New Bottom Plate_v1 (Autodesk Fusion 360 design; units mm, degrees)
Autodesk Fusion 360 part; units mm, degrees
sketch "Sketch1" plane through (0, 0, 0) normal (0, 0, 1) x (1, 0, 0)
  line L0 (0, 0) -> (342.375, 0)
  line L1 (342.375, 0) -> (342.375, 123.3)
  line L2 (342.375, 123.3) -> (0, 123.3)
  line L3 (0, 123.3) -> (0, 0)
  dimension "d1" = 342.375
  dimension "d2" = 123.3
  constraint horizontal L0
  constraint vertical L1
  constraint horizontal L2
  constraint vertical L3
  constraint coincident L0.start L3.end
  measures "d1" distance of L1.end L2.end
  measures "d2" distance of L0.start L2.end
extrude "Extrude1" add sketch "Sketch1" along normal blind 1
fillet "Fillet1" radius 2.5 4 edges at (0, 0, 0.5) (342.375, 0, 0.5) (342.375, 123.3, 0.5) (0, 123.3, 0.5)
sketch "Sketch2" plane through (0, 0, 1) normal (0, 0, 1) x (-1, 0, 0)
  arc A0 (-2.5, -123.3) -> (0, -120.8) centre (-2.5, -120.8) ccw
  line L0 (0, -120.8) -> (0, -2.5)
  arc A1 (0, -2.5) -> (-2.5, 0) centre (-2.5, -2.5) ccw
  line L1 (-2.5, 0) -> (-339.875, 0)
  arc A2 (-339.875, 0) -> (-342.375, -2.5) centre (-339.875, -2.5) ccw
  line L2 (-342.375, -2.5) -> (-342.375, -120.8)
  arc A3 (-342.375, -120.8) -> (-339.875, -123.3) centre (-339.875, -120.8) ccw
  line L3 (-339.875, -123.3) -> (-2.5, -123.3)
  line L4 (-5.5, -117.8) -> (-5.5, -5.5) construction
  line L5 (-5.5, -5.5) -> (-336.147, -5.5) construction
  line L6 (-5.5, -117.8) -> (-336.856, -117.8) construction
  line L7 (-336.147, -5.5) -> (-336.856, -117.8) construction
  line L8 (-336.147, -5.5) -> (-5.5, -117.8)
  line L9 (-5.5, -5.5) -> (-336.856, -117.8)
  line L10 (-5.9, -117.1907) -> (-5.9, -117.4)
  line L11 (-7.5002, -117.4) -> (-5.9, -117.4)
  line L12 (-8, -5.9) -> (-5.9, -5.9)
  line L13 (-5.9, -117.1907) -> (-5.9, -5.9)
  line L14 (-5.9, 0) -> (-5.9, 15)
  line L15 (-7.5002, -117.4) -> (-335.747, -117.4)
  line L16 (-8, -5.9) -> (-335.747, -5.9)
  line L17 (-335.747, -5.9) -> (-335.747, -117.4242)
  dimension "d7" = 5.5
  dimension "d8" = 5.5
  dimension "d9" = 5.5
  dimension "d10" = 6.228
  dimension "d11" = 5.519
  dimension "d16" = 0.4
  dimension "d17" = 0.4
  dimension "d18" = 0.4
  constraint vertical L4
  constraint perpendicular L4 L5
  constraint perpendicular L4 L6
  constraint perpendicular L6 L10
  constraint perpendicular L1 L13
  constraint perpendicular L4 L12
  constraint coincident L1 L14.start
  constraint collinear L13 L14
  constraint perpendicular L2 L15
  constraint coincident L9 L17.end
  measures "d7" distance of L1 L4.end
  measures "d8" distance of L0 L4.end
  measures "d9" distance of L3 L4.start
  measures "d10" distance of L2 L5.end
  measures "d11" distance of L2 L6.end
  measures "d16" distance of L4 L13
  measures "d17" distance of L5 L12
  measures "d18" distance of L6 L11
extrude "Extrude2" add sketch "Sketch2" along normal blind 2 contours L8 L9 L12 L16 | L8 L9 L15 L16 L17 | L8 L9 L10 L11 L12 L13 | L8 L9 L11 L15
sketch "Sketch3" plane through (0, 0, 1) normal (0, 0, 1) x (-1, 0, 0)
  line L0 (-5.9, -5.9) -> (-5.9, -117.4)
  line L1 (-5.9, -117.4) -> (-335.747, -117.4)
  line L2 (-335.747, -117.4) -> (-335.747, -5.9)
  line L3 (-335.747, -5.9) -> (-5.9, -5.9)
  arc A0 (-2.5, -123.3) -> (0, -120.8) centre (-2.5, -120.8) ccw
  line L4 (0, -120.8) -> (0, -2.5)
  arc A1 (0, -2.5) -> (-2.5, 0) centre (-2.5, -2.5) ccw
  line L5 (-2.5, 0) -> (-339.875, 0)
  arc A2 (-339.875, 0) -> (-342.375, -2.5) centre (-339.875, -2.5) ccw
  line L6 (-342.375, -2.5) -> (-342.375, -120.8)
  arc A3 (-342.375, -120.8) -> (-339.875, -123.3) centre (-339.875, -120.8) ccw
  line L7 (-339.875, -123.3) -> (-2.5, -123.3)
  line L8 (-6.2203, -99.9759) -> (-6.2199, -118.8)
  line L9 (-6.2246, -4.5) -> (-6.2082, -61.8661)
  line L10 (-6.2082, -61.8661) -> (-6.2095, -61.8663)
  line L11 (0.0269, -120.8) -> (-0.7247, -2.5)
  line L12 (-125.03, -5.5) -> (-14.265, -5.5)
  line L13 (-14.2649, -117.8) -> (-73.858, -117.8)
  line L14 (-14.265, -4.5) -> (-6.2246, -4.5)
  line L15 (-14.265, -5.5) -> (-6.2247, -5.5)
  line L16 (-14.2649, -117.8004) -> (-6.2199, -117.8002)
  arc A4 (-2.4783, -123.3004) -> (0.0269, -120.8) centre (-2.459, -120.8147) ccw
  line L17 (-6.2095, -61.8663) -> (-6.2054, -78.9217)
  line L18 (-133.07, -5.5) -> (-133.07, -4.5)
  line L19 (-73.858, -117.8) -> (-73.858, -118.8)
  line L20 (-81.898, -118.8) -> (-81.898, -117.8)
  arc A5 (-0.7247, -2.5) -> (-3.225, 0) centre (-3.2248, -2.5001) ccw
  line L21 (-332.837, -117.8) -> (-333.8375, -117.8)
  line L22 (-332.8375, -4) -> (-332.8375, -2.5)
  line L23 (-332.837, -4) -> (-310.8413, -4)
  line L24 (-73.858, -117.8003) -> (-73.858, -118.8)
  line L25 (-73.858, -118.8) -> (-81.898, -118.8)
  line L26 (-340.62, -123.2958) -> (-335.838, -123.3)
  line L27 (-81.898, -118.8) -> (-81.898, -117.8)
  line L28 (-332.837, -118.8) -> (-332.837, -117.8)
  line L29 (-333.8375, -118.8) -> (-333.838, -118.8)
  arc A6 (-343.1178, -120.7937) -> (-340.62, -123.2958) centre (-340.6178, -120.7958) ccw
  line L30 (-247.164, -117.8) -> (-324.797, -117.8)
  line L31 (-296.48, -4.5) -> (-296.48, -5.5)
  line L32 (-333.8375, -117.8) -> (-333.8375, -118.8)
  line L33 (-337.5995, -117.8) -> (-337.5995, -4)
  line L34 (-333.838, -117.8) -> (-337.5995, -117.8)
  line L35 (-247.164, -118.8) -> (-247.164, -117.8)
  line L36 (-324.797, -118.8) -> (-332.837, -118.8)
  line L37 (-333.838, -118.8) -> (-333.838, -117.8)
  line L38 (-324.797, -117.8) -> (-324.797, -118.8)
  line L39 (-3.225, 0) -> (-340.5995, 0)
  line L40 (-343.0995, -99.75) -> (-343.1178, -120.7937)
  line L41 (-6.2083, -80.9225) -> (-6.2049, -97.9745)
  line L42 (-6.2062, -99.9739) -> (-6.2203, -99.9759)
  line L43 (-6.2065, -80.9222) -> (-6.2083, -80.9225)
  line L44 (-310.8413, -4) -> (-310.8413, -5.5)
  line L45 (-343.0995, -2.5) -> (-343.0995, -99.75)
  arc A7 (-0.7247, -2.5) -> (-3.225, 0.0001) centre (-3.2248, -2.5001) ccw
  line L46 (-6.2054, -78.9217) -> (-6.207, -78.922)
  line L47 (-332.837, -2.5) -> (-332.837, -4)
  line L48 (-337.5995, -4) -> (-332.8375, -4)
  line L49 (-304.52, -5.5) -> (-304.52, -4.5)
  arc A8 (-340.5995, 0) -> (-343.0995, -2.5) centre (-340.5995, -2.5) ccw
  line L50 (-335.838, -123.3) -> (-2.4783, -123.3004)
  line L51 (-310.8413, -5.5) -> (-304.52, -5.5)
  line L52 (-6.2083, -61.8661) -> (-6.2095, -61.8663)
  line L53 (-304.52, -4.5) -> (-296.48, -4.5)
  line L54 (-296.48, -5.5) -> (-133.07, -5.5)
  line L55 (-332.8375, -2.5) -> (-332.837, -2.5)
  line L56 (-14.265, -5.5) -> (-14.265, -4.5)
  line L57 (-14.265, -4.5) -> (-6.225, -4.5)
  line L58 (-6.2095, -61.8663) -> (-6.2054, -78.9217)
  line L59 (-6.225, -4.5) -> (-6.2083, -61.8661)
  line L60 (-81.898, -117.8) -> (-239.124, -117.8)
  line L61 (-337.5995, -117.8) -> (-337.5995, -4)
  line L62 (-3.225, 0.0001) -> (-340.5995, 0)
  line L63 (-335.838, -123.3) -> (-2.4783, -123.3)
  line L64 (-247.164, -117.8) -> (-324.797, -117.8)
  line L65 (-296.48, -5.5) -> (-133.07, -5.5)
  line L66 (-14.2649, -117.8004) -> (-73.858, -117.8003)
  line L67 (-6.2203, -99.9759) -> (-6.2199, -118.8)
  line L68 (-6.2065, -80.9222) -> (-6.2083, -80.9225)
  line L69 (-6.207, -78.922) -> (-6.2065, -80.9222)
  line L70 (-6.2083, -80.9225) -> (-6.2049, -97.9745)
  line L71 (-6.2049, -97.9745) -> (-6.2066, -97.9748)
  line L72 (-6.2066, -97.9748) -> (-6.2062, -99.9739)
  line L73 (-14.2649, -118.8) -> (-14.2649, -117.8004)
  arc A9 (-2.4783, -123.3) -> (0.0217, -120.8) centre (-2.4626, -120.8157) ccw
  line L74 (-125.03, -5.5) -> (-14.265, -5.5)
  line L75 (-6.2199, -118.8) -> (-14.2649, -118.8)
  line L76 (0.0217, -120.8) -> (-0.7247, -2.5)
  line L77 (-6.2062, -99.9739) -> (-6.2203, -99.9759)
  line L78 (-247.164, -118.8) -> (-247.164, -117.8)
  line L79 (-239.124, -118.8) -> (-247.164, -118.8)
  line L80 (-333.838, -118.8) -> (-333.838, -117.8)
  line L81 (-310.8413, -4) -> (-310.8413, -5.5)
  line L82 (-333.8375, -118.8) -> (-333.838, -118.8)
  line L83 (-333.8375, -117.8) -> (-333.8375, -118.8)
  line L84 (-332.8375, -4) -> (-332.8375, -2.5)
  line L85 (-332.837, -4) -> (-310.8413, -4)
  line L86 (-332.837, -117.8) -> (-333.8375, -117.8)
  line L87 (-332.837, -118.8) -> (-332.837, -117.8)
  line L88 (-332.8375, -2.5) -> (-332.837, -2.5)
  line L89 (-324.797, -118.8) -> (-332.837, -118.8)
  line L90 (-239.124, -117.8) -> (-239.124, -118.8)
  line L91 (-324.797, -117.8) -> (-324.797, -118.8)
  line L92 (-333.838, -117.8) -> (-337.5995, -117.8)
  line L93 (-296.48, -4.5) -> (-296.48, -5.5)
  line L94 (-332.837, -2.5) -> (-332.837, -4)
  arc A10 (-343.1178, -120.7937) -> (-340.62, -123.2958) centre (-340.6178, -120.7958) ccw
  line L95 (-343.0995, -99.75) -> (-343.1178, -120.7937)
  line L96 (-343.0995, -2.5) -> (-343.0995, -99.75)
  line L97 (-304.52, -5.5) -> (-304.52, -4.5)
  line L98 (-337.5995, -4) -> (-332.8375, -4)
  line L99 (-310.8413, -5.5) -> (-304.52, -5.5)
  arc A11 (-340.5995, 0) -> (-343.0995, -2.5) centre (-340.5995, -2.5) ccw
  line L100 (-304.52, -4.5) -> (-296.48, -4.5)
  line L101 (-340.62, -123.2958) -> (-335.838, -123.3)
  line L102 (-6.2066, -97.9748) -> (-6.2062, -99.9739)
  line L103 (-6.2199, -118.8) -> (-14.2649, -118.8)
  line L104 (-14.2649, -118.8) -> (-14.2649, -117.8)
  line L105 (-6.2049, -97.9745) -> (-6.2066, -97.9748)
  line L106 (-6.207, -78.922) -> (-6.2065, -80.9222)
  line L107 (-6.2054, -78.9217) -> (-6.207, -78.922)
  line L108 (-14.265, -5.5) -> (-14.265, -4.5)
  line L109 (-125.03, -4.5) -> (-125.03, -5.5)
  line L110 (-73.858, -118.8) -> (-81.898, -118.8)
  line L111 (-125.03, -4.5) -> (-125.03, -5.5)
  line L112 (-133.07, -4.5) -> (-125.03, -4.5)
  line L113 (-81.898, -117.8) -> (-239.124, -117.8)
  line L114 (-239.124, -117.8) -> (-239.124, -118.8)
  line L115 (-239.124, -118.8) -> (-247.164, -118.8)
  line L116 (-133.07, -5.5) -> (-133.07, -4.5)
  line L117 (-133.07, -4.5) -> (-125.03, -4.5)
  point P0 (-304.5, -5.5)
  dimension "d22" = 5.5
  dimension "d23" = 5.5
  dimension "d24" = 6.2339
  dimension "d25" = 5.5125
  dimension "d26" = 5.5
  dimension "d27" = 6.2276
  dimension "d28" = 5.5188
  constraint coincident L16.start L66.start
  constraint perpendicular L8 L16
  constraint coincident L16.end L67
  constraint coincident L12.end L15.start
  constraint perpendicular L15 L56
  constraint coincident L15.end L59
  measures "d22" distance of L50 L66
  measures "d23" distance of L12 L39
  measures "d24" distance of L8.end L11
  measures "d25" distance of L9.start L11
  measures "d26" distance of L33 L45
  measures "d27" distance of L16.end L11
  measures "d28" distance of L15.end L76
equation "d1 = 337.375 mm + 2.5 mm + 2.5 mm"
equation "d2 = 118.3 mm + 2.5 mm + 2.5 mm"
